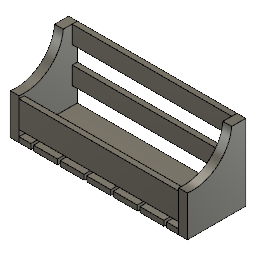
minibar v4 (Autodesk Fusion 360 design; units mm, degrees)
Autodesk Fusion 360 part; units mm, degrees
sketch "botn" plane through (0, 0, 0) normal (0, 1, 0) x (1, 0, 0)
  line L0 (450, -150) -> (-450, -150)
  line L1 (-450, -150) -> (-450, 150)
  line L2 (-450, 150) -> (450, 150)
  line L3 (450, 150) -> (450, -150)
  line L4 (450, -150) -> (-450, 150) construction
  line L5 (-450, -150) -> (450, 150) construction
  dimension "d11" = 900
  dimension "d12" = 300
  constraint horizontal L0
  constraint perpendicular L0 L1
  constraint parallel L0 L2
  constraint parallel L1 L3
  constraint coincident L4 origin
  constraint coincident L5 origin
  measures "d11" distance of L1.end L2.end
  measures "d12" distance of L0.start L2.end
extrude "Extrude1" add sketch "botn" along normal blind 30 makes body 1
sketch "Sketch2" plane through (0, 30, 0) normal (0, 1, 0) x (-1, 0, 0)
  line L0 (-450, -150) -> (450, -150)
  line L1 (450, -150) -> (450, 150)
  line L2 (450, 150) -> (-450, 150)
  line L3 (-450, 150) -> (-450, -150)
  line L4 (450, 150) -> (375, 150)
  line L5 (375, 150) -> (225, 150)
  line L6 (225, 150) -> (75, 150)
  line L7 (75, 150) -> (-75, 150)
  line L8 (-75, 150) -> (-225, 150)
  line L9 (-225, 150) -> (-375, 150)
  line L10 (-375, 150) -> (-450, 150)
  line L11 (225, 82.5) -> (225, 75)
  line L12 (75, 82.5) -> (75, 75)
  line L13 (-225, 82.5) -> (-225, 75)
  line L14 (-375, 82.5) -> (-375, 75)
  line L15 (217.5, 75) -> (217.5, 150)
  line L16 (217.5, 150) -> (232.5, 150)
  line L17 (232.5, 150) -> (232.5, 75)
  line L18 (232.5, 0) -> (217.5, 150) construction
  line L19 (217.5, 0) -> (232.5, 150) construction
  line L20 (67.5, 150) -> (82.5, 150)
  line L21 (82.5, 150) -> (82.5, 75)
  line L22 (67.5, 75) -> (67.5, 150)
  line L23 (67.5, 150) -> (82.5, 0) construction
  line L24 (82.5, 150) -> (74.2537, 67.5372) construction
  line L25 (-82.5, 150) -> (-67.5, 150)
  line L26 (-67.5, 150) -> (-67.5, 75)
  line L27 (-82.5, 75) -> (-82.5, 150)
  line L28 (-232.5, 150) -> (-217.5, 150)
  line L29 (-217.5, 150) -> (-217.5, 75)
  line L30 (-232.5, 75) -> (-232.5, 150)
  line L31 (-232.5, 150) -> (-217.5, 0) construction
  line L32 (-224.2537, 82.4628) -> (-232.5, 0) construction
  line L33 (-382.5, 150) -> (-367.5, 150)
  line L34 (-367.5, 150) -> (-367.5, 75)
  line L35 (-382.5, 75) -> (-382.5, 150)
  line L36 (-382.5, 150) -> (-374.2537, 67.5372) construction
  line L37 (-367.5, 150) -> (-382.5, 0) construction
  line L38 (367.5, 150) -> (367.5, 75)
  line L39 (382.5, 75) -> (382.5, 150)
  arc A0 (367.5, 75) -> (382.5, 75) centre (375, 75) ccw
  arc A1 (217.5, 75) -> (232.5, 75) centre (225, 75) ccw
  arc A2 (225.7463, 82.4628) -> (224.2537, 82.4628) centre (225, 75) ccw
  arc A3 (67.5, 75) -> (82.5, 75) centre (75, 75) ccw
  arc A4 (75.7463, 82.4628) -> (74.2537, 82.4628) centre (75, 75) ccw
  arc A5 (-74.2537, 67.5372) -> (-67.5, 75) centre (-75, 75) ccw
  line L40 (-74.2537, 67.5372) -> (-67.5, 0) construction
  arc A6 (-82.5, 75) -> (-75.7463, 67.5372) centre (-75, 75) ccw
  arc A7 (-232.5, 75) -> (-217.5, 75) centre (-225, 75) ccw
  arc A8 (-224.2537, 82.4628) -> (-225.7463, 82.4628) centre (-225, 75) ccw
  arc A9 (-382.5, 75) -> (-367.5, 75) centre (-375, 75) ccw
  arc A10 (-374.2537, 82.4628) -> (-375.7463, 82.4628) centre (-375, 75) ccw
  line L41 (-67.5, 150) -> (-82.5, 150)
  line L42 (-67.5, 150) -> (-82.5, 150)
  line L43 (-74.2537, 82.4628) -> (-75, 75) construction
  line L44 (-75.7463, 67.5372) -> (-82.5, 0) construction
  arc A11 (-82.5, 75) -> (-74.2537, 67.5372) centre (-75, 75) ccw
  point P0 (225, 75)
  point P1 (75, 75)
  point P2 (-75, 75)
  point P3 (-225, 75)
  point P4 (-375, 75)
  dimension "d15" = 75
  dimension "d16" = 75
  dimension "d17" = 150
  dimension "d18" = 150
  dimension "d19" = 150
  dimension "d20" = 150
  dimension "d21" = 150
  dimension "d22" = 75
  dimension "d23" = 75
  dimension "d24" = 75
  dimension "d25" = 75
  dimension "d26" = 75
  dimension "d28" = 15
  dimension "d29" = 15
  dimension "d30" = 15
  dimension "d31" = 15
  dimension "d32" = 15
  dimension "d33" = 15
  dimension "d34" = 15
  dimension "d35" = 150
  dimension "d37" = 15
  dimension "d38" = 15
  constraint coincident L1.end L2.start
  constraint coincident L2 L4.end
  constraint perpendicular L1 L4
  constraint coincident L2 L5.end
  constraint coincident L2 L6.end
  constraint coincident L2 L7.end
  constraint parallel L2 L7
  constraint coincident L2 L8.end
  constraint coincident L2 L9.end
  constraint coincident L2.end L3.start
  constraint perpendicular L5 L11
  constraint perpendicular L6 L12
  constraint perpendicular L9 L13
  constraint perpendicular L10 L14
  constraint coincident P0 L11.end
  constraint coincident P1 L12.end
  constraint coincident P2 A5.centre
  constraint coincident P3 L13.end
  constraint coincident P4 L14.end
  constraint parallel L15 L17
  constraint coincident L18 P0
  constraint coincident L19 P0
  constraint horizontal L20
  constraint perpendicular L20 L21
  constraint parallel L21 L22
  constraint coincident L23 P1
  constraint coincident L24 P1
  constraint horizontal L25
  constraint perpendicular L25 L26
  constraint parallel L26 L27
  constraint coincident P2 L43
  constraint horizontal L28
  constraint perpendicular L28 L29
  constraint parallel L29 L30
  constraint coincident L31 P3
  constraint coincident L32 P3
  constraint horizontal L33
  constraint perpendicular L33 L34
  constraint parallel L34 L35
  constraint coincident L36 P4
  constraint coincident L37 P4
  constraint vertical L38
  constraint vertical L39
  constraint coincident L2 L39.end
  constraint coincident L18 A2.end
  constraint coincident L19 A2.start
  constraint concentric A1 A2
  constraint coincident L24.end A3
  constraint coincident L23 A4.end
  constraint coincident L24 A4.start
  constraint concentric A3 A4
  constraint coincident L27.start A5
  constraint coincident A6.end L43
  constraint coincident A4 L12.start
  constraint coincident A2 L11.start
  constraint coincident L32.start A7
  constraint coincident L31 A8.end
  constraint concentric A7 A8
  constraint coincident A8 L13.start
  constraint coincident L36.end A9
  constraint coincident L36 A10.end
  constraint coincident L14.start A9
  constraint coincident L37 A10.start
  constraint concentric A9 A10
  constraint collinear L43 L44
  measures "d15" distance of L1.end L4.end
  measures "d16" distance of L4.end A0.centre
  measures "d17" distance of L4.end L5.end
  measures "d18" distance of L5.end L6.end
  measures "d19" distance of L6.end L7.end
  measures "d20" distance of L7.end L8.end
  measures "d21" distance of L8.end L9.end
  measures "d22" distance of L5.end P0
  measures "d23" distance of L6.end P1
  measures "d24" distance of L7.end P2
  measures "d25" distance of L8.end P3
  measures "d26" distance of L9.end P4
  measures "d28" diameter of A0
  measures "d29" diameter of A1
  measures "d30" diameter of A3
  measures "d31" diameter of A5
  measures "d32" diameter of A7
  measures "d33" diameter of A9
  measures "d34" distance of L15.end L16.end
  measures "d35" distance of L19.start L15.end
  measures "d37" distance of L40.end L44.end
  measures "d38" distance of L31.end L32.end
extrude "Extrude2" cut sketch "Sketch2" against normal blind 30 contours L2 L9 L10 L33 L34 L35 A9 | L2 L4 L5 L38 L39 A0 | L2 L8 L9 L28 L29 L30 A7 | L2 L5 L6 L15 L16 L17 A1 | L2 L7 L8 L25 L26 L27 A5 A6 L41 L42 A11 | L2 L6 L7 L20 L21 L22 A3 bodies 1
sketch "Hlid1" plane through (-450, 0, 0) normal (-1, 0, 0) x (0, 0, 1)
  line L0 (-150, 0) -> (150, 0)
  line L1 (150, 0) -> (150, 30)
  line L2 (150, 30) -> (-150, 30)
  line L3 (-150, 30) -> (-150, 0)
  line L4 (150, 0) -> (-150, 0)
  line L5 (-150, 0) -> (-150, 430)
  line L6 (-150, 430) -> (-100, 430)
  line L7 (150, 230) -> (150, 0)
  line L8 (-150, 430) -> (-100, 430)
  line L9 (150, 0) -> (150, 230)
  arc A0 (-100, 430) -> (150, 230) centre (119.2359, 447.7948) ccw
  dimension "d45" = 300
  dimension "d47" = 50
  dimension "d48" = 230
  dimension "d51" = 430
  constraint horizontal L4
  constraint vertical L5
  constraint horizontal L6
  constraint vertical L7
  constraint coincident L0.end L1.start
  constraint perpendicular L5 L8
  measures "d45" distance of L0.end L0.start
  measures "d47" distance of L5.end L6.end
  measures "d48" distance of L0.end L7.start
  measures "d51" distance of L0.start L5.end
extrude "Extrude3" add sketch "Hlid1" along normal blind 50 separate body makes body 2
sketch "Hlid 2" plane through (450, 0, 0) normal (1, 0, 0) x (0, 0, -1)
  line L0 (-150, 0) -> (150, 0)
  line L1 (150, 0) -> (150, 30)
  line L2 (150, 30) -> (-150, 30)
  line L3 (-150, 30) -> (-150, 0)
  line L4 (-150, 0) -> (150, 0)
  line L5 (150, 0) -> (150, 430)
  line L6 (150, 430) -> (-150, 430)
  line L7 (-150, 430) -> (-150, 0)
  line L8 (-150, 0) -> (-150, 230)
  line L9 (150, 430) -> (100, 430)
  arc A0 (-150, 230) -> (100, 430) centre (-121.125, 450.1562) ccw
  dimension "d52" = 430
  dimension "d53" = 300
  dimension "d54" = 230
  dimension "d55" = 50
  constraint horizontal L4
  constraint vertical L5
  constraint horizontal L6
  constraint vertical L7
  constraint coincident L0.start L3.end
  constraint perpendicular L4 L8
  constraint coincident L6 L9.end
  measures "d52" distance of L0.start L6.end
  measures "d53" distance of L0.start L0.end
  measures "d54" distance of L0.start L8.end
  measures "d55" distance of L5.end L9.end
extrude "Extrude4" add sketch "Hlid 2" along normal blind 50 separate body contours L0 L1 L2 L3 L4 L5 L7 L8 | L2 L5 L6 L7 L8 L9 A0 makes body 3
form "Form1" [no effect]
sketch "lenging" plane through (0, 30, 0) normal (0, 1, 0) x (-1, 0, 0)
  line L0 (-82.5, 75) -> (-82.5, 150)
  line L1 (-82.5, 150) -> (-217.5, 150)
  line L2 (-217.5, 150) -> (-217.5, 75)
  arc A0 (-232.5, 75) -> (-217.5, 75) centre (-225, 75) ccw
  line L3 (-232.5, 75) -> (-232.5, 150)
  line L4 (-232.5, 150) -> (-367.5, 150)
  line L5 (-367.5, 150) -> (-367.5, 75)
  arc A1 (-382.5, 75) -> (-367.5, 75) centre (-375, 75) ccw
  line L6 (-382.5, 75) -> (-382.5, 150)
  line L7 (-382.5, 150) -> (-450, 150)
  line L8 (-450, 150) -> (-450, -150)
  line L9 (-450, -150) -> (450, -150)
  line L10 (450, -150) -> (450, 150)
  line L11 (450, 150) -> (382.5, 150)
  line L12 (382.5, 150) -> (382.5, 75)
  arc A2 (367.5, 75) -> (382.5, 75) centre (375, 75) ccw
  line L13 (367.5, 75) -> (367.5, 150)
  line L14 (367.5, 150) -> (232.5, 150)
  line L15 (232.5, 150) -> (232.5, 75)
  arc A3 (217.5, 75) -> (232.5, 75) centre (225, 75) ccw
  line L16 (217.5, 75) -> (217.5, 150)
  line L17 (217.5, 150) -> (82.5, 150)
  line L18 (82.5, 150) -> (82.5, 75)
  arc A4 (67.5, 75) -> (82.5, 75) centre (75, 75) ccw
  line L19 (67.5, 75) -> (67.5, 150)
  line L20 (67.5, 150) -> (-67.5, 150)
  line L21 (-67.5, 150) -> (-67.5, 75)
  arc A5 (-82.5, 75) -> (-67.5, 75) centre (-75, 75) ccw
  line L22 (450, -150) -> (-450, -150)
  line L23 (-450, -150) -> (-450, -180)
  line L24 (-450, -180) -> (450, -180)
  line L25 (450, -180) -> (450, -150)
  dimension "d58" = 30
  constraint perpendicular L22 L23
  constraint parallel L22 L24
  constraint parallel L23 L25
  constraint coincident L8.end L9.start
  constraint perpendicular L8 L22
  constraint coincident L9.end L10.start
  measures "d58" distance of L9.end L24.end
extrude "Extrude5" add sketch "lenging" against normal blind 30 contours L9 L22 L23 L24 L25 bodies 1
sketch "lenging 2" plane through (0, 430, 0) normal (0, 1, 0) x (-1, 0, 0)
  line L0 (-450, -150) -> (-450, -100)
  line L1 (-450, -100) -> (-500, -100)
  line L2 (-500, -100) -> (-500, -150)
  line L3 (-500, -150) -> (-450, -150)
  line L4 (-500, -150) -> (-450, -150)
  line L5 (-450, -150) -> (-450, -180)
  line L6 (-450, -180) -> (-500, -180)
  line L7 (-500, -180) -> (-500, -150)
  line L8 (450, -150) -> (500, -150)
  line L9 (500, -150) -> (500, -180)
  line L10 (500, -180) -> (450, -180)
  line L11 (450, -180) -> (450, -150)
  dimension "d61" = 30
  dimension "d62" = 50
  dimension "d63" = 30
  dimension "d64" = 50
  constraint horizontal L4
  constraint vertical L5
  constraint horizontal L6
  constraint vertical L7
  constraint coincident L2.end L3.start
  constraint horizontal L8
  constraint vertical L9
  constraint horizontal L10
  constraint vertical L11
  measures "d61" distance of L2.end L6.end
  measures "d62" distance of L8.start L8.end
  measures "d63" distance of L8.start L10.end
  measures "d64" distance of L2.end L0.start
extrude "Extrude6" add sketch "lenging 2" against normal blind 430 contours L3 L4 L5 L6 L7 | L8 L9 L10 L11 bodies 2 3
sketch "Sketch8" plane through (450, 0, 0) normal (-1, 0, 0) x (0, 0, 1)
  line L0 (-180, 0) -> (150, 0)
  line L1 (150, 0) -> (150, 230)
  arc A0 (-100, 430) -> (150, 230) centre (121.125, 450.1562) ccw
  line L2 (-100, 430) -> (-180, 430)
  line L3 (-180, 430) -> (-180, 0)
  line L4 (-180, 430) -> (-150, 430)
  line L5 (-150, 430) -> (-150, 330)
  line L6 (-150, 330) -> (-180, 330)
  line L7 (-180, 330) -> (-180, 430)
  line L8 (-180, 330) -> (-150, 330)
  line L9 (-150, 330) -> (-150, 230)
  line L10 (-150, 230) -> (-180, 230)
  line L11 (-180, 230) -> (-180, 330)
  line L12 (-180, 230) -> (-150, 230)
  line L13 (-150, 230) -> (-150, 130)
  line L14 (-150, 130) -> (-180, 130)
  line L15 (-180, 130) -> (-180, 230)
  dimension "d67" = 30
  dimension "d68" = 100
  dimension "d69" = 30
  dimension "d70" = 100
  dimension "d71" = 30
  dimension "d72" = 100
  constraint horizontal L4
  constraint vertical L5
  constraint horizontal L6
  constraint vertical L7
  constraint coincident L2.end L3.start
  constraint horizontal L8
  constraint vertical L9
  constraint horizontal L10
  constraint vertical L11
  constraint horizontal L12
  constraint vertical L13
  constraint horizontal L14
  constraint vertical L15
  measures "d67" distance of L2.end L4.end
  measures "d68" distance of L2.end L6.end
  measures "d69" distance of L6.end L5.end
  measures "d70" distance of L6.end L10.end
  measures "d71" distance of L10.end L9.end
  measures "d72" distance of L10.end L14.end
extrude "Extrude7" add sketch "Sketch8" along normal blind 900 separate body contours L3 L10 L12 L13 L14 L15 | L2 L3 L4 L5 L6 L7 L8 makes body 4 at (150, 396.6667, -180) makes body 5 at (150, 196.6667, -180)
sketch "Sketch9" plane through (450, 0, 0) normal (-1, 0, 0) x (0, 0, 1)
  line L0 (-180, 0) -> (150, 0)
  line L1 (150, 0) -> (150, 230)
  arc A0 (-100, 430) -> (150, 230) centre (121.125, 450.1562) ccw
  line L2 (-100, 430) -> (-180, 430)
  line L3 (-180, 430) -> (-180, 0)
  line L4 (150, 230) -> (120, 230)
  line L5 (120, 230) -> (120, 215)
  line L6 (120, 215) -> (150, 215)
  line L7 (150, 215) -> (150, 230)
  line L8 (120, 215) -> (150, 215)
  line L9 (150, 215) -> (150, 65)
  line L10 (150, 65) -> (120, 65)
  line L11 (120, 65) -> (120, 215)
  dimension "d75" = 30
  dimension "d76" = 15
  dimension "d77" = 30
  dimension "d78" = 150
  constraint horizontal L4
  constraint vertical L5
  constraint horizontal L6
  constraint vertical L7
  constraint coincident L1.end A0.end
  constraint horizontal L8
  constraint vertical L9
  constraint horizontal L10
  constraint vertical L11
  measures "d75" distance of L1.end L4.end
  measures "d76" distance of L1.end L6.end
  measures "d77" distance of L5.end L6.end
  measures "d78" distance of L5.end L10.end
extrude "Extrude8" add sketch "Sketch9" along normal blind 900 separate body contours L1 L6 L8 L9 L10 L11 makes body 6
equation "b_l = 900 mm"
equation "fjoldi_g = 6"
equation "fjar_g = ( b_l / fjoldi_g ) / 2"
equation "b_b = 300 mm"
equation "h1 = 400 mm"
equation "h2 = 200 mm"
equation "þykkt_hlid = 50 mm"
equation "þykkt_rest = 30 mm"
equation "h_spyta = 100 mm"
equation "h_framan = 150 mm"
equation "d11 = b_l"
equation "d12 = b_b"
equation "d13 = þykkt_rest"
equation "d15 = fjar_g"
equation "d16 = b_b / 4"
equation "d17 = fjar_g * 2"
equation "d18 = fjar_g * 2"
equation "d19 = fjar_g * 2"
equation "d20 = fjar_g * 2"
equation "d21 = fjar_g * 2"
equation "d22 = b_b / 4"
equation "d23 = b_b / 4"
equation "d24 = b_b / 4"
equation "d25 = b_b / 4"
equation "d26 = b_b / 4"
equation "þykkt_g = 15 mm"
equation "d28 = þykkt_g"
equation "d29 = þykkt_g"
equation "d30 = þykkt_g"
equation "d31 = þykkt_g"
equation "d32 = þykkt_g"
equation "d33 = þykkt_g"
equation "d34 = þykkt_g"
equation "d35 = b_b / 2"
equation "d37 = þykkt_g"
equation "d38 = þykkt_g"
equation "d43 = -þykkt_rest"
equation "d45 = b_b"
equation "d47 = þykkt_hlid"
equation "d48 = h2 + þykkt_rest"
equation "d49 = þykkt_hlid"
equation "d51 = h1 + þykkt_rest"
equation "d52 = h1 + þykkt_rest"
equation "d53 = b_b"
equation "d54 = h2 + þykkt_rest"
equation "d55 = þykkt_hlid"
equation "d56 = þykkt_hlid"
equation "d58 = þykkt_rest"
equation "d59 = -þykkt_rest"
equation "d61 = þykkt_rest"
equation "d62 = þykkt_hlid"
equation "d63 = þykkt_rest"
equation "d65 = -( h1 + þykkt_rest )"
equation "d67 = þykkt_rest"
equation "d68 = h_spyta"
equation "d69 = þykkt_rest"
equation "d70 = h_spyta"
equation "d71 = þykkt_rest"
equation "d72 = h_spyta"
equation "d73 = b_l"
equation "d75 = þykkt_rest"
equation "d76 = þykkt_g"
equation "d77 = þykkt_rest"
equation "d78 = h_framan"
equation "d79 = b_l"
named bodies: "Botn", "Hlið 1", "Hlid 2", "aftan1", "aftan 2", "framan"
